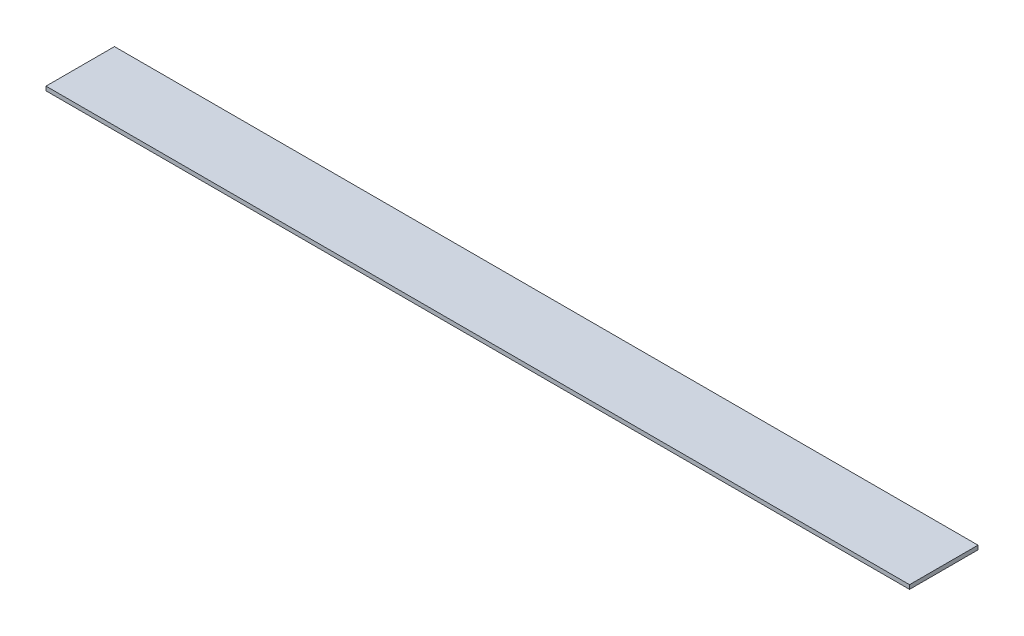
# Autodesk Inventor part: MSC 0562 rib cone
Saved by Autodesk Inventor 2025 (Build 290162010, 162A)
## iProperties
Created: 2024-06-26
Part Number: MSC 0562 rib cone
Material: Stainless Steel
Document SubType Name: Sheet Metal
Designer: pokla
Density: 8 g/cm^3
Sheet Metal Rule: AISI304 3mm Die 32
Appearance: Default
Author: pokla
Autodesk Inventor part; units mm, degrees
ref_plane "YZ Plane" through (0, 0, 0) normal (1, 0, 0) x (0, 1, 0)
ref_plane "XZ Plane" through (0, 0, 0) normal (0, 1, 0) x (-1, 0, 0)
ref_plane "XY Plane" through (0, 0, 0) normal (0, 0, 1) x (1, 0, 0)
sketch "Sketch1" plane through (0, 0, 0) normal (0, 0, 1) x (1, 0, 0)
  line L0 (190, 758.8462) -> (190, 378.8462) construction
  line L1 (190, 378.8462) -> (190, 159.8058) construction
  line L2 (190, 758.8462) -> (190, 1137.6923) construction
  line L3 (98.5795, 0) -> (749.422, 1137.6923) construction
  line L4 (570, 1137.6923) -> (570, 824.0572) construction
  line L5 (190, 758.8462) -> (532.6945, 758.8462) construction
  line L6 (190, 378.8462) -> (315.307, 378.8462)
  line L7 (-190, 758.8462) -> (-532.6945, 758.8462) construction
  line L8 (-190, 758.8462) -> (-190, 1137.6923) construction
  line L9 (-571.5, 826.6793) -> (-568.5, 821.4352) construction
  line L10 (-570, 1137.6923) -> (-570, 824.0572) construction
  line L11 (-749.422, 1137.6923) -> (749.422, 1137.6923) construction
  line L12 (-190, 758.8462) -> (190, 758.8462) construction
  line L13 (190, 378.8462) -> (-190, 378.8462)
  line L14 (-190, 378.8462) -> (-190, 758.8462) construction
  line L15 (-190, 378.8462) -> (-190, 159.8058) construction
  line L16 (-98.5795, 0) -> (98.5795, 0) construction
  line L17 (0, 1137.6923) -> (0, 0) construction
  line L18 (-98.5795, 0) -> (-749.422, 1137.6923) construction
  line L19 (-190, 378.8462) -> (-315.307, 378.8462)
  point P0 (0, 758.8462)
  point P1 (0, 568.8462)
  point P2 (-190, 568.8462)
  dimension "d0" = 1498.844
  dimension "d1" = 197.159
  dimension "d2" = 1310.702
  dimension "d3" = 380
  dimension "d4" = 380
  dimension "d5" = 380
  dimension "d6" = 380
  measures "d0" distance of L11.start L3.end
  measures "d1" distance of L18.start L3.start
  measures "d2" distance of L3.start L3.end
  measures "d3" distance of L1.start L13.end
  measures "d4" distance of L0.start L1.start
  measures "d5" distance between parallel lines of L8 L10
  measures "d6" distance between parallel lines of L2 L4
contour flange "Contour Flange1" sketch "Sketch1" thickness 3 bend radius 5 width 50 along (0, 0, 1) mid plane no both sides yes wall seen from (252.6535, 378.8462, 0) lies toward (0, 1, 0) curves L6 L13 L19
bend "Bend1"
corner "Corner1"
equation "\"d5\" = d3"
equation "\"d6\" = d3"
equation "\"d7\" = Thickness"
equation "\"d8\" = BendReliefWidth"
equation "\"d9\" = BendReliefDepth"
equation "\"d10\" = MinimumRemnant"
equation "\"d11\" = TransitionRadius"
equation "\"d13\" = BendRadius"
equation "\"d15\" = CornerReliefSize"
equation "\"d16\" = GapSize"
equation "\"d17\" = JacobiRadiusSize"
equation "\"BendReliefWidth\" = Thickness"
equation "\"BendReliefDepth\" = 0.5 * Thickness"
equation "\"CornerReliefSize\" = 4 * Thickness"
equation "\"MinimumRemnant\" = 2 * Thickness"
equation "\"TransitionRadius\" = BendRadius"
equation "\"JacobiRadiusSize\" = BendRadius"
equation "\"GapSize\" = Thickness"
equation "\"Thickness\" = 3"
equation "\"BendRadius\" = 5"
body "Solid1"
